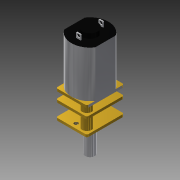
# Autodesk Inventor part: micro motor pololu
Saved by Autodesk Inventor 2016 (Build 200138000, 138)
## iProperties
Created: 2013-12-20
Part Number: micro motor pololu
Material: Generic
Document SubType Name: Modeling
Designer: JustinIndra
Density: 1 g/cm^3
Appearance: Default
Author: JustinIndra
Autodesk Inventor part; units mm, degrees
ref_plane "YZ Plane" through (0, 0, 0) normal (1, 0, 0) x (0, 1, 0)
ref_plane "XZ Plane" through (0, 0, 0) normal (0, 1, 0) x (-1, 0, 0)
sketch "Sketch1" plane through (0, 0, 0) normal (0, 0, 1) x (1, 0, 0)
  circle A0 centre (0, 0) radius 6
  line L0 (-5, 3.3166) -> (-5, -3.3166)
  line L1 (5, 3.3166) -> (5, -3.3166)
  dimension "d0" = 12
  dimension "d1" = 10
  constraints: 4 end point, 4 point on circle, 2 parallel, 1 centre point, 1 coincident, 1 vertical
  measures "d0" diameter of A0
  measures "d1" distance between parallel lines of L1 L0
extrude "Extrusion1" add sketch "Sketch1" along normal blind 15 contours L1 A0 L0
sketch "Sketch2" plane through (0, 0, 15) normal (0, 0, 1) x (1, 0, 0)
  arc A0 (5, 3.3166) -> (-5, 3.3166) centre (0, 0) ccw projected
  circle A1 centre (0, 0) radius 2.5
  dimension "d4" = 5
  constraints: 1 centre point, 1 coincident
  measures "d4" diameter of A1
extrude "Extrusion2" add sketch "Sketch2" along normal blind 1.5
sketch "Sketch3" plane through (0, 0, 15) normal (0, 0, 1) x (1, 0, 0)
  circle A0 centre (0, 0) radius 2.5 projected
  line L0 (-0.775, 3.775) -> (0.775, 3.775)
  line L1 (0.775, 3.775) -> (0.775, 3.475)
  line L2 (0.775, 3.475) -> (-0.775, 3.475)
  line L3 (-0.775, 3.475) -> (-0.775, 3.775)
  point P0 (0, 3.475)
  dimension "d7" = 3.775
  dimension "d8" = 0.3
  dimension "d9" = 1.55
  constraints: 8 end point, 2 parallel, 1 horizontal, 1 midpoint, 1 perpendicular, 1 vertical alignment
  measures "d7" distance from line of A0.centre L0
  measures "d8" distance of L0.end L1.end
  measures "d9" distance of L0.start L0.end
extrude "Extrusion3" add sketch "Sketch3" along normal blind 1.65 contours L0 L1 L2 L3
sketch "Sketch4" plane through (-0.775, 3.775, 15) normal (0, 1, 0) x (1, 0, 0)
  line L0 (1.55, -1.65) -> (0, -1.65) projected
  circle A0 centre (0.775, -0.95) radius 0.5
  point P0 (0.775, 15)
  point P1 (0.775, -1.65)
  dimension "d12" = 1
  dimension "d13" = 0.7
  constraints: 1 centre point, 1 midpoint, 1 vertical alignment
  measures "d12" diameter of A0
  measures "d13" distance from line of L0 A0.centre
extrude "Extrusion4" cut sketch "Sketch4" against normal up to surface (0.3 mm away)
fillet "Fillet1" radius 0.25 2 edges at (0.775, 3.625, 16.65) (-0.775, 3.625, 16.65)
mirror "Mirror1" about plane through (0, 0, 0) normal (0, 1, 0) of "Extrusion3", "Extrusion4", "Fillet1"
sketch "Sketch5" plane through (0, 0, 0) normal (0, 0, -1) x (-1, 0, 0)
  arc A0 (5, 3.3166) -> (-5, 3.3166) centre (0, 0) ccw projected
  line L0 (-5, -3.3166) -> (-5, 3.3166) projected
  line L1 (-5, 6) -> (5, 6)
  line L2 (5, 6) -> (5, -6)
  line L3 (5, -6) -> (-5, -6)
  line L4 (-5, -6) -> (-5, 6)
  point P0 (0, 6)
  point P1 (-5, 0)
  constraints: 8 end point, 2 midpoint, 2 parallel, 1 collinear, 1 horizontal, 1 horizontal alignment, 1 perpendicular, 1 tangent, 1 vertical alignment
extrude "Extrusion5" add sketch "Sketch5" along normal blind 0.8
sketch "Sketch6" plane through (0, 0, -0.8) normal (0, 0, -1) x (-1, 0, 0)
  line L0 (5, 6) -> (-5, 6) projected
  line L1 (-5, 6) -> (-5, -6) projected
  line L2 (-5, -6) -> (5, -6) projected
  line L3 (5, -6) -> (5, 6) projected
  circle A0 centre (2.85, 3.85) radius 1.5
  circle A1 centre (-2.85, -3.85) radius 1.5
  point P0 (0, 0)
  dimension "d19" = 3
  dimension "d20" = 2.15
  dimension "d21" = 2.15
  dimension "d22" = 3
  dimension "d23" = 2.15
  dimension "d24" = 2.15
  constraints: 2 centre point
  measures "d19" diameter of A0
  measures "d20" distance from line of L3 A0.centre
  measures "d21" distance from line of L0 A0.centre
  measures "d22" diameter of A1
  measures "d23" distance from line of L1 A1.centre
  measures "d24" distance from line of L2 A1.centre
extrude "Extrusion6" add sketch "Sketch6" along normal blind 8.2 contours A0 | A1
ref_plane "Work Plane1" through (0, 0, -3.15) normal (0, 0, -1) x (-1, 0, 0)
sketch "Sketch7" plane through (0, 0, -3.15) normal (0, 0, -1) x (-1, 0, 0)
  line L0 (-5, 6) -> (5, 6)
  line L1 (5, 6) -> (5, -6)
  line L2 (5, -6) -> (-5, -6)
  line L3 (-5, -6) -> (-5, 6)
  line L4 (-5, 6) -> (-5, -6) projected
  line L5 (5, -6) -> (5, 6) projected
  line L6 (5, 6) -> (-5, 6) projected
  line L7 (-5, -6) -> (5, -6) projected
  point P0 (0, 0)
  constraints: 8 end point, 4 collinear, 2 parallel, 1 horizontal, 1 perpendicular
extrude "Extrusion7" add sketch "Sketch7" along normal blind 0.8
sketch "Sketch8" plane through (-2.85, 3.85, -9) normal (0, 0, -1) x (-1, 0, 0)
  line L0 (-7.85, 2.15) -> (2.15, 2.15)
  line L1 (2.15, 2.15) -> (2.15, -9.85)
  line L2 (2.15, -9.85) -> (-7.85, -9.85)
  line L3 (-7.85, -9.85) -> (-7.85, 2.15)
  line L4 (2.15, -9.85) -> (2.15, 2.15) projected
  line L5 (2.15, 2.15) -> (-7.85, 2.15) projected
  line L6 (-7.85, 2.15) -> (-7.85, -9.85) projected
  line L7 (-7.85, -9.85) -> (2.15, -9.85) projected
  point P0 (-2.85, -3.85)
  constraints: 8 end point, 4 collinear, 2 parallel, 1 horizontal, 1 perpendicular
extrude "Extrusion8" add sketch "Sketch8" against normal blind 0.8
sketch "Sketch9" plane through (0, 0, -9) normal (0, 0, -1) x (-1, 0, 0)
  point P0 (0, 0)
  point P1 (0, 4.5)
  point P2 (0, -4.5)
  dimension "d32" = 4.5
  dimension "d33" = 4.5
  constraints: 2 vertical alignment
  measures "d32" distance of point (0, 0) point (0, 4.5)
  measures "d33" distance of point (0, 0) point (0, -4.5)
hole "Hole1" at (0, 4.5, -9) at (0, -4.5, -9) direction (0, 0, 1) diameter 1.221 depth 1 thread size "M1.6x0.35" class "6H" standard "ISO Metric profile"
sketch "Sketch10" plane through (0, 0, -9) normal (0, 0, -1) x (-1, 0, 0)
  circle A0 centre (0, 0) radius 1.95
  dimension "d41" = 3.9
  constraints: 1 centre point, 1 coincident
  measures "d41" diameter of A0
extrude "Extrusion9" add sketch "Sketch10" along normal blind 0.6
sketch "Sketch11" plane through (0, 0, -9.6) normal (0, 0, -1) x (-1, 0, 0)
  circle A0 centre (0, 0) radius 1.95 projected
  circle A1 centre (0, 0) radius 1.5
  line L0 (-1.118, 1) -> (1.118, 1)
  dimension "d44" = 3
  dimension "d45" = 1
  constraints: 2 end point, 2 point on circle, 1 centre point, 1 coincident, 1 horizontal
  measures "d44" diameter of A1
  measures "d45" distance from line of A1.centre L0
extrude "Extrusion10" add sketch "Sketch11" along normal blind 9.27 contours A1 L0 picked at (0.0594, 0.1702)
fillet "Fillet2" radius 0.5 1 edges at (1.95, 0, -9.6)
fillet "Fillet3" radius 0.5 12 edges at (5, -6, -8.6) (5, 6, -8.6) (-5, -6, -8.6) (-5, 6, -8.6) (-5, 6, -3.55) (-5, 6, -0.4) (-5, -6, -3.55) (-5, -6, -0.4) (5, -6, -0.4) (5, -6, -3.55) (5, 6, -3.55) (5, 6, -0.4)
equation "\"d33\" = d32"
body "Solid1"
